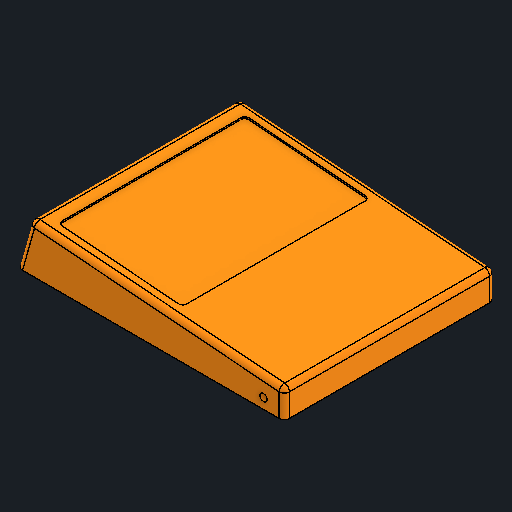
# Autodesk Inventor part: Pedal
Saved by Autodesk Inventor 2026.2 (Build 302298000, 298)
## iProperties
Created: 2015-05-05
Part Number: Pedal
Material: Steel, Cast
Document SubType Name: Modeling
Designer: Philip
Density: 7.85 g/cm^3
Appearance: Orange
Author: Philip
Autodesk Inventor part; units mm, degrees
ref_plane "YZ Plane" through (0, 0, 0) normal (1, 0, 0) x (0, 1, 0)
ref_plane "XZ Plane" through (0, 0, 0) normal (0, 1, 0) x (-1, 0, 0)
ref_plane "XY Plane" through (0, 0, 0) normal (0, 0, 1) x (1, 0, 0)
sketch "Sketch1" plane through (0, 0, 0) normal (0, 0, 1) x (1, 0, 0)
  line L0 (0, 0) -> (-81.661, 0)
  line L1 (-81.661, 0) -> (-77.5429, 14.6731)
  line L2 (-77.5429, 14.6731) -> (0, 8.509)
  line L3 (0, 8.509) -> (0, 0)
  dimension "d0" = 81.661
  dimension "d1" = 15.24
  dimension "d2" = 77.7875
  dimension "d3" = 8.509
  constraints: 8 end point, 1 horizontal, 1 perpendicular
  measures "d0" distance of L0.start L0.end
  measures "d1" distance of L0.end L1.end
  measures "d2" distance of L1.end L2.end
  measures "d3" distance of L2.end L0.start
extrude "Extrusion1" add sketch "Sketch1" along normal mid plane 64.389
fillet "Fillet1" radius 1.5875 8 edges at (-38.7714, 11.591, 32.1945) (0, 8.509, 0) (0, 4.2545, 32.1945) (0, 4.2545, -32.1945) (-38.7714, 11.591, -32.1945) (-77.5429, 14.6731, 0) (-79.6019, 7.3365, -32.1945) (-79.6019, 7.3365, 32.1945)
shell "Shell1" thickness 1.905 removed faces 1 at (-53.8706, 0, 10.7315)
sketch "Sketch3" plane through (-1.4617, 8.6252, 30.607) normal (0.0792423, 0.9968554, 0) x (0.9968554, -0.0792423, 0)
  line L0 (-33.3933, 2.032) -> (-71.4933, 2.032)
  line L1 (-71.4933, 2.032) -> (-71.4933, 59.182)
  line L2 (-71.4933, 59.182) -> (-33.3933, 59.182)
  line L3 (-33.3933, 59.182) -> (-33.3933, 2.032)
  line L4 (-75.0156, 0) -> (-75.0156, 61.214) projected
  line L5 (-76.5733, 61.214) -> (-76.5733, 0) projected
  line L6 (2.1406, 30.607) -> (-92.8395, 30.607)
  point P0 (-71.4933, 30.607)
  dimension "d8" = 57.15
  dimension "d9" = 38.1
  dimension "d11" = 5.08
  constraints: 10 end point, 2 horizontal, 2 parallel, 1 midpoint, 1 perpendicular, 1 point on line
  measures "d8" distance of L2.end L0.start
  measures "d9" distance of L1.end L2.end
  measures "d11" distance between parallel lines of L5 L1
extrude "Extrusion2" cut sketch "Sketch3" against normal blind 0.508
fillet "Fillet2" radius 1.27 4 edges at (-34.7702, 11.0172, -28.575) (-72.7503, 14.0363, -28.575) (-72.7503, 14.0363, 28.575) (-34.7702, 11.0172, 28.575)
sketch "Sketch4" plane through (-77.8957, 13.4161, -30.607) normal (-0.9627994, 0.2702173, 0) x (0, 0, 1)
  line L0 (61.214, -13.9344) -> (0, -13.9344) projected
  line L1 (30.607, -13.9344) -> (30.607, -2.8384)
  point P0 (30.607, 8.1318)
  point P1 (30.607, -9.7434)
  dimension "d15" = 4.191
  constraints: 2 end point, 1 midpoint, 1 point on line, 1 vertical
  measures "d15" distance from line of L0 point (30.607, -9.743)
hole "Hole1" at (-80.5285, 4.0351, 0) direction (0.9627994, -0.2702173, 0) diameter 2.159 end through all
sketch "Sketch5" plane through (0, 0, -32.1945) normal (0, 0, -1) x (-1, 0, 0)
  line L0 (0, 7.0427) -> (0, 0) projected
  line L1 (1.5875, 0) -> (80.0122, 0) projected
  point P0 (6.35, 3.175)
  dimension "d23" = 6.35
  dimension "d24" = 3.175
  measures "d23" distance from line of L0 point (6.35, 3.175)
  measures "d24" distance from line of L1 point (6.35, 3.175)
hole "Hole2" at (-6.35, 3.175, -32.1945) direction (0, 0, 1) diameter 2.159 end through all
body "Solid1"
